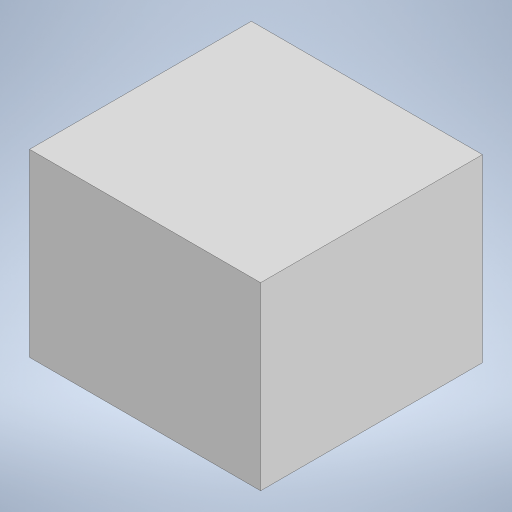
# Autodesk Inventor part: guide_base
Saved by Autodesk Inventor 2023.5 (Build 275446000, 446)
## iProperties
Created: 2025-03-29
Part Number: guide_base
Material: 常规
Document SubType Name: Modeling
Designer: jiaxue
Density: 1 g/cm^3
Appearance: 默认
Author: jiaxue
Autodesk Inventor part; units mm, degrees
ref_plane "YZ Plane" through (0, 0, 0) normal (1, 0, 0) x (0, 1, 0)
ref_plane "XZ Plane" through (0, 0, 0) normal (0, 1, 0) x (-1, 0, 0)
ref_plane "XY Plane" through (0, 0, 0) normal (0, 0, 1) x (1, 0, 0)
sketch "草图1" plane through (0, 0, 0) normal (1, 0, 0) x (0, 1, 0)
  line L0 (-19.5, -24) -> (19.5, -24)
  line L1 (19.5, -24) -> (19.5, 24)
  line L2 (19.5, 24) -> (-19.5, 24)
  line L3 (-19.5, 24) -> (-19.5, -24)
  line L4 (-19.5, -24) -> (19.5, 24) construction
  line L5 (19.5, -24) -> (-19.5, 24) construction
  point P0 (0, 0)
  dimension "d0" = 39
  dimension "d1" = 48
  constraints: 12 end point, 2 midpoint, 2 parallel, 1 horizontal, 1 perpendicular
  measures "d0" distance of L2.end L1.end
  measures "d1" distance of L1.end L0.end
extrude "拉伸1" add sketch "草图1" against normal blind 50
